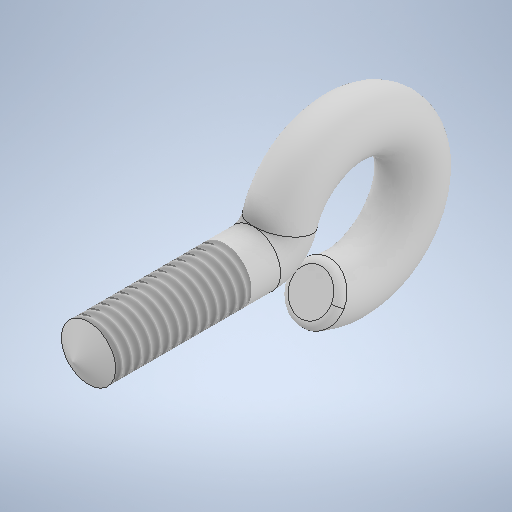
# Autodesk Inventor part: HookScrew
Saved by Autodesk Inventor 2025 (Build 290162000, 162)
## iProperties
Created: 2024-06-19
Part Number: HookScrew
Material: Generic
Document SubType Name: Modeling
Designer: mumin
Density: 1 g/cm^3
Appearance: Default
Author: mumin
Autodesk Inventor part; units mm, degrees
ref_plane "YZ Plane" through (0, 0, 0) normal (1, 0, 0) x (0, 1, 0)
ref_plane "XZ Plane" through (0, 0, 0) normal (0, 1, 0) x (-1, 0, 0)
ref_plane "XY Plane" through (0, 0, 0) normal (0, 0, 1) x (1, 0, 0)
sketch "Sketch1" plane through (0, 0, 0) normal (1, 0, 0) x (0, 1, 0)
  line L0 (0, 0) -> (0, -13.2918)
  line L1 (0, 0) -> (13.2918, 0) construction
  arc A0 (-4.3301, -17.5) -> (1.4286, -15.2084) centre (0, -20) ccw
  line L2 (0, -20) -> (-4.3301, -17.5) construction
  line L3 (0, -20) -> (0, -15) construction
  arc A1 (0, -13.2918) -> (1.4286, -15.2084) centre (2, -13.2918) ccw
  dimension "d0" = 15
  dimension "d1" = 90
  dimension "d2" = 60
  dimension "d3" = 5
  dimension "d4" = 2
  constraints: 8 end point, 5 point on circle, 2 centre point, 2 tangent, 1 coincident, 1 horizontal, 1 perpendicular, 1 point on line, 1 vertical
  measures "d0" distance of L0.start L3.end
  measures "d1" angle of L0 L1
  measures "d2" angle of L3 L2
  measures "d3" distance of L3.end L2.start
  measures "d4" radius of A1
sketch "Sketch2" plane through (0, 0, 0) normal (0, 0, 1) x (1, 0, 0)
  circle A0 centre (0, 0) radius 2
  dimension "d5" = 4
  constraints: 1 centre point, 1 coincident
  measures "d5" diameter of A0
sweep "Sweep1" add profiles "Sketch2" path "Sketch1" path curves L0 A1 A0
sketch "Sketch3" plane through (0, 0, 0) normal (1, 0, 0) x (0, 1, 0)
  line L0 (0, 0) -> (2, -1.1547)
  line L1 (0, 0) -> (2.3094, 0) construction
  line L2 (2, -1.1547) -> (2, 0)
  line L3 (2, 0) -> (-2, 0) projected
  line L4 (2, 0) -> (0, 0)
  line L5 (2, 0) -> (2, -4.8576) construction
  line L6 (0, 1.6102) -> (0, -2.3094) construction
  dimension "d8" = 30
  constraints: 12 end point, 2 perpendicular, 2 vertical, 1 equal length, 1 horizontal, 1 point on line
  measures "d8" angle of L0 L1
revolve "Revolution1" cut sketch "Sketch3" angle 360 about axis through (0, 0, 1.6102) along (0, 0, -1)
thread "Thread1"
fillet "Fillet1" radius 0.5 1 edges at (-2, -4.3301, -17.5)
body "Solid1"
